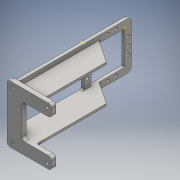
# Autodesk Inventor part: hold
Saved by Autodesk Inventor 2016 (Build 200138000, 138)
## iProperties
Created: 2023-04-16
Part Number: hold
Material: 常规
Document SubType Name: Modeling
Designer: Administrator
Density: 1 g/cm^3
Appearance: 默认
Author: Administrator
Autodesk Inventor part; units mm, degrees
ref_plane "YZ Plane" through (0, 0, 0) normal (1, 0, 0) x (0, 1, 0)
ref_plane "XZ Plane" through (0, 0, 0) normal (0, 1, 0) x (-1, 0, 0)
ref_plane "XY Plane" through (0, 0, 0) normal (0, 0, 1) x (1, 0, 0)
sketch "草图1" plane through (0, 0, 0) normal (1, 0, 0) x (0, 1, 0)
  point P0 (0, 0)
sketch "草图2" plane through (0, 0, 0) normal (1, 0, 0) x (0, 1, 0)
  line L0 (0, 0) -> (32, 0)
  line L1 (32, 0) -> (32, -32)
  line L2 (32, -32) -> (0, -32)
  line L3 (0, -32) -> (0, 0)
  line L4 (4.7, -4.7) -> (27.4, -4.7)
  line L5 (27.4, -4.7) -> (27.4, -27.4)
  line L6 (27.4, -27.4) -> (4.7, -27.4)
  line L7 (4.7, -27.4) -> (4.7, -4.7)
  dimension "d0" = 32
  dimension "d1" = 32
  dimension "d2" = 22.7
  dimension "d3" = 22.7
  constraints: 16 end point, 4 parallel, 2 horizontal, 2 perpendicular
  measures "d0" distance of L1.end L2.end
  measures "d1" distance of L0.end L1.end
  measures "d2" distance of L5.end L6.end
  measures "d3" distance of L4.end L5.end
extrude "拉伸1" add sketch "草图2" along normal blind 2
sketch "草图3" plane through (2, 0, 0) normal (1, 0, 0) x (0, 0, -1)
  point P0 (4.7, 27.4)
  point P1 (4.7, 4.7)
hole "孔1" at (2, 29.65, -16) direction (-1, 0, 0) diameter 2 end through all
sketch "草图4" plane through (2, 0, 0) normal (1, 0, 0) x (0, 0, -1)
  point P0 (0, 0)
sketch "草图5" plane through (2, 0, 0) normal (1, 0, 0) x (0, 0, -1)
  point P0 (0, 0)
hole "孔2" at (2, 2.35, -16) direction (-1, 0, 0) diameter 2 end through all
hole "孔3" at (2, 16, -2.35) direction (-1, 0, 0) diameter 2 end through all
hole "孔4" at (2, 16, -29.65) direction (-1, 0, 0) diameter 2 end through all
hole "孔5" at (2, 29.65, -10.6) direction (-1, 0, 0) diameter 2 end through all
hole "孔6" at (2, 29.65, -21.5) direction (-1, 0, 0) diameter 2 end through all
hole "孔7" at (2, 21.5, -2.35) direction (-1, 0, 0) diameter 2 end through all
hole "孔8" at (2, 10.6, -2.35) direction (-1, 0, 0) diameter 2 end through all
hole "孔9" at (2, 21.5, -29.65) direction (-1, 0, 0) diameter 2 end through all
hole "孔10" at (2, 10.6, -29.65) direction (-1, 0, 0) diameter 2 end through all
hole "孔11" at (2, 2.35, -10.6) direction (-1, 0, 0) diameter 2 end through all
hole "孔12" at (2, 2.35, -21.5) direction (-1, 0, 0) diameter 2 end through all
sketch "草图6" plane through (2, 0, 0) normal (1, 0, 0) x (0, 0, -1)
  circle A0 centre (2.35, 10.6) radius 1 projected
  circle A1 centre (2.35, 10.6) radius 1
  circle A2 centre (29.65, 10.6) radius 1 projected
  circle A3 centre (29.65, 10.6) radius 1
  point P0 (0, 0)
  constraints: 2 centre point, 2 coincident
extrude "拉伸2" add sketch "草图6" against normal blind 2
sketch "草图8" plane through (0, 0, -32) normal (0, -1, 0) x (1, 0, 0)
  point P0 (0, 32)
sketch "草图9" plane through (0, 0, 0) normal (0, 0, 1) x (1, 0, 0)
  point P0 (0, 0)
sketch "草图10" plane through (2, 27.4, -4.7) normal (0, 0, -1) x (-1, 0, 0)
  line L0 (0, -27.4) -> (-15, -27.4)
  line L1 (2, -27.4) -> (2, 4.6) projected
  line L2 (0, -27.4) -> (0, -17.4)
  line L3 (0, -22.7) -> (0, 0) projected
  line L4 (0, -17.4) -> (-15, -27.4)
  dimension "d121" = 15
  dimension "d123" = 10
  constraints: 6 end point, 1 horizontal, 1 point on line
  measures "d121" distance of L0.start L0.end
  measures "d123" distance of L0.start L2.end
sketch "草图11" plane through (0, 4.7, -27.4) normal (0, 0, 1) x (1, 0, 0)
  line L0 (2, -4.7) -> (2, 5.3)
  line L1 (2, 22.7) -> (2, 0) projected
  line L2 (2, -4.7) -> (17, -4.7)
  line L3 (17, -4.7) -> (2, 5.3)
  point P0 (0, -4.7)
  dimension "d124" = 10
  dimension "d125" = 15
  constraints: 6 end point, 1 horizontal, 1 point on line
  measures "d124" distance of L0.start L0.end
  measures "d125" distance of L0.start L2.end
sketch "草图12" plane through (0, 0, -32) normal (0, -1, 0) x (1, 0, 0)
  point P0 (0, 32)
extrude "拉伸3" add sketch "草图10" against normal blind 1.5
extrude "拉伸4" add sketch "草图11" against normal blind 1.5
sketch "草图13" plane through (0, 0, -32) normal (0, -1, 0) x (1, 0, 0)
  line L0 (0, 0) -> (2, 0) projected
  line L1 (0, 0) -> (2, 0)
  line L2 (17, 3.1) -> (17, 4.6)
  line L3 (2, 27.3) -> (17, 27.3)
  line L4 (2, 28.8) -> (17, 28.8) projected
  line L5 (17, 27.3) -> (17, 28.8)
  line L6 (17, 28.8) -> (2, 28.8)
  line L7 (2, 28.8) -> (2, 32)
  line L8 (2, 27.3) -> (17, 27.3) projected
  line L9 (17, 28.8) -> (17, 27.3)
  line L10 (17, 27.3) -> (0, 27.3)
  line L11 (0, 32) -> (2, 32)
  line L12 (2, 30.65) -> (2, 28.65) projected
  line L13 (2, 32) -> (2, 28.65)
  line L14 (0, 0) -> (2, 0)
  line L15 (0, 32) -> (0, 27.3)
  line L16 (0, 0) -> (0, 32) projected
  line L17 (17, 4.6) -> (2, 4.6) projected
  line L18 (17, 4.6) -> (0, 4.6)
  line L19 (0, 0) -> (0, 4.6)
  line L20 (0, 0) -> (2, 0)
  line L21 (2, 3.1) -> (2, 0) projected
  line L22 (17, 4.6) -> (17, 3.1) projected
  line L23 (2, 3.1) -> (17, 3.1)
  constraints: 32 end point, 6 perpendicular, 2 collinear, 2 horizontal, 2 point on line, 1 vertical
extrude "拉伸5" add sketch "草图13" along normal blind 50
sketch "草图14" plane through (0, -50, -32) normal (0, -1, 0) x (1, 0, 0)
  line L0 (30, 29.3) -> (30, 33.3)
  line L1 (28, 35.3) -> (2, 35.3)
  line L2 (30, 2.6) -> (30, -1.4)
  line L3 (28, -3.4) -> (2, -3.4)
  line L4 (10, 25.3) -> (10, 6.6)
  line L5 (28, 27.3) -> (12, 27.3)
  line L6 (28, 4.6) -> (12, 4.6)
  arc A0 (12, 27.3) -> (10, 25.3) centre (12, 25.3) ccw
  arc A1 (2, 35.3) -> (0, 33.3) centre (2, 33.3) ccw
  arc A2 (30, 33.3) -> (28, 35.3) centre (28, 33.3) ccw
  arc A3 (28, 27.3) -> (30, 29.3) centre (28, 29.3) ccw
  arc A4 (30, 2.6) -> (28, 4.6) centre (28, 2.6) ccw
  arc A5 (28, -3.4) -> (30, -1.4) centre (28, -1.4) ccw
  arc A6 (0, -1.4) -> (2, -3.4) centre (2, -1.4) ccw
  arc A7 (10, 6.6) -> (12, 4.6) centre (12, 6.6) ccw
  circle A8 centre (27, 32.3) radius 1
  circle A9 centre (27, -0.4) radius 1
  circle A10 centre (3, 32.3) radius 1
  circle A11 centre (3, -0.4) radius 1
  line L7 (0, 33.3) -> (0, -1.4)
  circle A12 centre (27, -0.4) radius 1
  circle A13 centre (27, 32.3) radius 1
  point P0 (0, 32)
  point P1 (30, 27.3)
  point P2 (0, 4.6)
  point P3 (30, 4.6)
  point P4 (10, 4.6)
  dimension "d146" = 2
  dimension "d149" = 2
  dimension "d152" = 2
  dimension "d154" = 2
  constraints: 16 end point, 16 point on circle, 14 centre point, 14 tangent, 8 equal radius, 6 point on line, 2 coincident, 1 horizontal, 1 perpendicular, 1 vertical
  measures "d146" diameter of A8
  measures "d149" diameter of A9
  measures "d152" diameter of A10
  measures "d154" diameter of A11
extrude "拉伸6" add sketch "草图14" against normal blind 3
fillet "圆角1" radius 3 1 edges at (1, 32, 0)
fillet "圆角2" radius 3 1 edges at (1, 32, -32)
sketch "草图15" plane through (0, -47, -32) normal (0, 1, 0) x (1, 0, 0)
  circle A0 centre (3, -32.3) radius 1 projected
  circle A1 centre (3, -32.3) radius 1
  circle A2 centre (3, 0.4) radius 1 projected
  circle A3 centre (3, 0.4) radius 1
  point P0 (0, -32)
  constraints: 2 centre point, 2 coincident
extrude "拉伸7" add sketch "草图15" against normal blind 3
sketch "草图16" plane through (0, -47, -32) normal (0, 1, 0) x (1, 0, 0)
  line L0 (0, -35.3) -> (4, -35.3)
  line L1 (2, -35.3) -> (28, -35.3) projected
  line L2 (4, -35.3) -> (1, -35.3)
  line L3 (4, -35.3) -> (4, -32.3)
  line L4 (28, 3.4) -> (2, 3.4) projected
  line L5 (0, 3.4) -> (4, 3.4)
  line L6 (4, 3.4) -> (4, 0.4)
  circle A0 centre (4, -32.3) radius 1
  circle A1 centre (4, 0.4) radius 1
  point P0 (0, -32)
  dimension "d161" = 4
  dimension "d163" = 3
  dimension "d166" = 4
  dimension "d167" = 3
  dimension "d168" = 2
  dimension "d169" = 2
  constraints: 10 end point, 3 point on line, 2 centre point, 2 coincident, 1 perpendicular, 1 vertical
  measures "d161" distance of L0.start L0.end
  measures "d163" distance of L0.end L3.end
  measures "d166" distance of L5.start L5.end
  measures "d167" distance of L5.end L6.end
  measures "d168" diameter of A0
  measures "d169" diameter of A1
extrude "拉伸8" cut sketch "草图16" against normal blind 3
fillet "圆角3" radius 1 1 edges at (2, 10, -3.95)
fillet "圆角4" radius 1 1 edges at (2, 10, -28.15)
fillet "圆角5" radius 1 1 edges at (17, 0, -3.95)
fillet "圆角6" radius 1 1 edges at (17, 0, -28.15)
fillet "圆角7" radius 1 1 edges at (17, -47, -3.95)
fillet "圆角8" radius 1 1 edges at (17, -47, -28.15)
fillet "圆角9" radius 1 1 edges at (1, 0, -27.4)
fillet "圆角10" radius 1 1 edges at (1, 0, -4.7)
sketch "草图17" plane through (2, 0, 0) normal (1, 0, 0) x (0, 0, -1)
  point P0 (0, 0)
sketch "草图18" plane through (0, 0, -26.4) normal (0, -1, 0) x (1, 0, 0)
  point P0 (0, 26.4)
